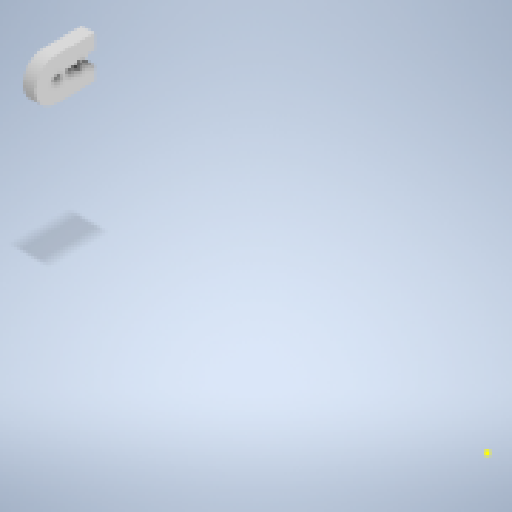
# Autodesk Inventor part: Крепление рычага к лицу
Saved by Autodesk Inventor 2023.2 (Build 272271030, 271C)
## iProperties
Created: 2024-02-06
Part Number: Крепление рычага к лицу
Material: Типовые
Document SubType Name: Modeling
Designer: I9232
Density: 1 g/cm^3
Appearance: По умолчанию
Author: I9232
Autodesk Inventor part; units mm, degrees
ref_plane "YZ Plane" through (0, 0, 0) normal (1, 0, 0) x (0, 1, 0)
ref_plane "XZ Plane" through (0, 0, 0) normal (0, 1, 0) x (-1, 0, 0)
ref_plane "XY Plane" through (0, 0, 0) normal (0, 0, 1) x (1, 0, 0)
sketch "Эскиз1" plane through (0, 0, 0) normal (0, 0, 1) x (1, 0, 0)
  line L0 (-186.8805, 58.4127) -> (-192.8805, 58.4127)
  line L1 (-192.8805, 58.4127) -> (-192.8805, 78.4127)
  line L2 (-192.8805, 78.4127) -> (-186.8805, 78.4127)
  line L3 (-186.8805, 78.4127) -> (-186.8805, 58.4127)
  line L4 (-192.8805, 65.9127) -> (-192.8805, 70.9127) projected
  point P0 (0, 0)
  point P1 (-192.8805, 68.4127)
  dimension "d0" = 20
  dimension "d1" = 6
  dimension "d19" = 0
  constraints: 8 end point, 2 parallel, 1 horizontal, 1 midpoint, 1 perpendicular
  measures "d0" distance of L0.end L1.end
  measures "d1" distance of L1.end L2.end
  measures "d19" distance from line of point (-192.881, 68.413) L1
extrude "Выдавливание1" add sketch "Эскиз1" along normal blind 25
fillet "Сопряжение1" radius 10 2 edges at (-189.8805, 58.4127, 25) (-189.8805, 78.4127, 25)
sketch "Эскиз2" plane through (-192.8805, 58.4127, 0) normal (-1, 0, 0) x (0, 0, 1)
  circle A0 centre (15, 10) radius 1.9
  line L0 (0, 20) -> (0, 0) projected
  line L1 (0, 10) -> (25, 10) construction
  arc A1 (15, 0) -> (15, 20) centre (15, 10) ccw projected
  point P0 (0, -58.4127)
  dimension "d5" = 3.8
  constraints: 2 end point, 1 centre point, 1 coincident, 1 horizontal, 1 midpoint, 1 point on circle
  measures "d5" diameter of A0
extrude "Выдавливание2" cut sketch "Эскиз2" against normal up to surface (6 mm away)
sketch "Эскиз3" plane through (0, 0, 0) normal (0, 0, -1) x (-1, 0, 0)
  line L0 (192.8805, 58.4127) -> (186.8805, 58.4127)
  line L1 (186.8805, 58.4127) -> (186.8805, 65.4127)
  line L2 (186.8805, 65.4127) -> (192.8805, 65.4127)
  line L3 (192.8805, 65.4127) -> (192.8805, 58.4127)
  line L4 (186.8805, 78.4127) -> (192.8805, 78.4127) projected
  line L5 (186.8805, 78.4127) -> (192.8805, 78.4127)
  line L6 (192.8805, 78.4127) -> (192.8805, 71.4127)
  line L7 (192.8805, 71.4127) -> (186.8805, 71.4127)
  line L8 (186.8805, 71.4127) -> (186.8805, 78.4127)
  point P0 (0, 0)
  dimension "d8" = 7
  dimension "d9" = 7
  dimension "d18" = 6
  constraints: 16 end point, 4 parallel, 2 horizontal, 2 perpendicular, 1 point on line
  measures "d8" distance of L0.end L1.end
  measures "d9" distance of L7.end L4.start
  measures "d18" distance of L0.start L0.end
extrude "Выдавливание3" add sketch "Эскиз3" along normal blind 2
sketch "Эскиз4" plane through (-192.8805, 68.4127, 15) normal (-1, 0, 0) x (0, 0, 1)
  line L0 (-15, 3) -> (-15, -3) projected
  line L1 (-15, 0) -> (-4.7, 0)
  line L2 (-4.7, 0) -> (-4.7, -1.5)
  line L3 (-15, -1.5) -> (-15, 0)
  line L4 (-4.7, 0) -> (-4.7, 1.5)
  line L5 (-10.2565, 0) -> (-12.2169, 0)
  line L6 (-11.5169, -1.5) -> (-11.5169, -2.7)
  line L7 (-11.5169, -2.7) -> (-9.7169, -2.7)
  line L8 (-9.7169, -2.7) -> (-9.7169, -1.5)
  line L9 (-11.5169, 1.5) -> (-11.5169, 2.7)
  line L10 (-11.5169, 2.7) -> (-9.7169, 2.7)
  line L11 (-9.7169, 2.7) -> (-9.7169, 1.5)
  line L12 (-4.7, -1.5) -> (-9.7169, -1.5)
  line L13 (-11.5169, -1.5) -> (-15, -1.5)
  line L14 (-4.7, 1.5) -> (-9.7169, 1.5)
  line L15 (-11.5169, 1.5) -> (-15, 1.5)
  line L16 (-4.7, 1.5) -> (-9.7169, 1.5)
  line L17 (-11.5169, 1.5) -> (-15, 1.5)
  point P0 (-15, -68.4127)
  dimension "d12" = 10.3
  dimension "d13" = 1.5
  dimension "d16" = 1.8
  dimension "d17" = 5.4
  constraints: 34 end point, 5 parallel, 4 symmetric about line, 2 horizontal, 2 perpendicular, 1 midpoint, 1 point on line
  measures "d12" distance of L2.end L3.start
  measures "d13" distance of L1.end L2.end
  measures "d16" distance of L6.end L7.end
  measures "d17" distance of L11.start L7.end
extrude "Выдавливание4" cut sketch "Эскиз4" against normal up to surface (6 mm away)
sketch "Эскиз5" plane through (0, 0, -2) normal (0, 0, -1) x (-1, 0, 0)
  point P0 (0, 0)
sketch "Эскиз6" plane through (0, 0, -2) normal (0, 0, -1) x (-1, 0, 0)
  line L0 (186.8805, 71.4127) -> (192.8805, 71.4127)
  line L1 (192.8805, 71.4127) -> (192.8805, 78.4127)
  line L2 (192.8805, 78.4127) -> (186.8805, 78.4127)
  line L3 (186.8805, 78.4127) -> (186.8805, 71.4127)
  line L4 (192.8805, 65.4127) -> (186.8805, 65.4127)
  line L5 (186.8805, 65.4127) -> (186.8805, 58.4127)
  line L6 (186.8805, 58.4127) -> (192.8805, 58.4127)
  line L7 (192.8805, 58.4127) -> (192.8805, 65.4127)
  point P0 (0, 0)
  constraints: 16 end point
sketch "Эскиз7" plane through (0, 0, -2) normal (0, 0, -1) x (-1, 0, 0)
  point P0 (0, 0)
extrude "Выдавливание5" add sketch "Эскиз6" along normal blind 1
